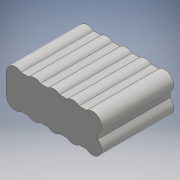
# Autodesk Inventor part: NimhBattery
Saved by Autodesk Inventor 2016 (Build 200138000, 138)
## iProperties
Created: 2016-02-21
Part Number: NimhBattery
Material: Generic
Document SubType Name: Modeling
Designer: jmurdo3
Density: 1 g/cm^3
Appearance: Default
Author: jmurdo3
Autodesk Inventor part; units mm, degrees
ref_plane "YZ Plane" through (0, 0, 0) normal (1, 0, 0) x (0, 1, 0)
ref_plane "XZ Plane" through (0, 0, 0) normal (0, 1, 0) x (-1, 0, 0)
ref_plane "XY Plane" through (0, 0, 0) normal (0, 0, 1) x (1, 0, 0)
sketch "Sketch1" plane through (0, 0, 0) normal (0, 1, 0) x (-1, 0, 0)
  circle A0 centre (0, 0) radius 9
  circle A1 centre (-19.25, 0) radius 9
  circle A2 centre (-38.5, 0) radius 9
  circle A3 centre (19.25, 0) radius 9
  circle A4 centre (38.5, 0) radius 9
  circle A5 centre (0, -20) radius 9
  circle A6 centre (-19.25, -20) radius 9
  circle A7 centre (-38.5, -20) radius 9
  circle A8 centre (19.25, -20) radius 9
  circle A9 centre (38.5, -20) radius 9
  line L0 (47.5, -20) -> (47.5, 0)
  line L1 (32.6799, -26.8648) -> (25.0701, -26.8648)
  line L2 (13.4299, -26.8648) -> (5.8201, -26.8648)
  line L3 (-5.8201, -26.8648) -> (-13.4299, -26.8648)
  line L4 (-25.0701, -26.8648) -> (-32.6799, -26.8648)
  line L5 (-32.6799, 6.8648) -> (-25.0701, 6.8648)
  line L6 (-13.4299, 6.8648) -> (-5.8201, 6.8648)
  line L7 (5.8201, 6.8648) -> (13.4299, 6.8648)
  line L8 (25.0701, 6.8648) -> (32.6799, 6.8648)
  line L9 (-43.8129, -12.7355) -> (-43.8129, -7.2645)
  dimension "d0" = 18
  dimension "d1" = 18
  dimension "d2" = 18
  dimension "d3" = 18
  dimension "d4" = 18
  dimension "d5" = 1.25
  dimension "d6" = 1.25
  dimension "d7" = 1.25
  dimension "d8" = 1.25
  dimension "d9" = 18
  dimension "d10" = 2
  dimension "d11" = 18
  dimension "d12" = 18
  dimension "d13" = 18
  dimension "d14" = 18
  dimension "d15" = 2
  dimension "d16" = 1.25
  dimension "d17" = 1.25
  dimension "d18" = 1.25
  dimension "d19" = 1.25
  dimension "d20" = 2
  dimension "d21" = 2
  constraints: 20 end point, 20 point on circle, 16 parallel, 10 centre point, 4 perpendicular, 2 tangent, 1 coincident, 1 vertical
  measures "d0" diameter of A0
  measures "d1" diameter of A1
  measures "d2" diameter of A2
  measures "d3" diameter of A3
  measures "d4" diameter of A4
  measures "d9" diameter of A5
  measures "d11" diameter of A6
  measures "d12" diameter of A7
  measures "d13" diameter of A8
  measures "d14" diameter of A9
extrude "Extrusion1" add sketch "Sketch1" along normal blind 72
body "Solid1"
